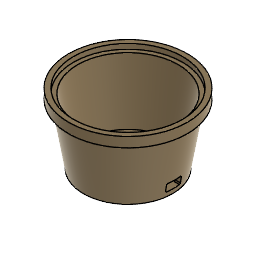
pot bottom v2 (Autodesk Fusion 360 design; units mm, degrees)
Autodesk Fusion 360 part; units mm, degrees
sketch "Sketch1" plane through (0, 0, 0) normal (0, 1, 0) x (1, 0, 0)
  line L0 (0, 0) -> (0, -70)
  line L1 (0, -70) -> (60, -70)
  line L2 (60, -70) -> (60, -60)
  line L3 (60, -60) -> (55, -60)
  line L4 (55, -60) -> (45, 0)
  line L5 (45, 0) -> (0, 0)
  dimension "d1" = 90
  dimension "d2" = 70
  dimension "d3" = 45
  dimension "d4" = 60
  dimension "d5" = 5
  dimension "d6" = 10
  constraint coincident L0.start L5.end
  constraint vertical L0
  constraint perpendicular L0 L1
  constraint perpendicular L1 L2
  constraint perpendicular L2 L3
  measures "d1" angle of L0 L5
  measures "d2" distance of L0.start L0.end
  measures "d3" distance of L0.start L4.end
  measures "d4" distance of L0.end L1.end
  measures "d5" distance of L2.end L3.end
  measures "d6" distance of L1.end L2.end
revolve "Revolve1" add sketch "Sketch1" angle 360 about axis through (0, 0, 0) along (0, 0, 1)
shell "Shell1" thickness 5 removed faces 1 at (28.282, -12.1475, 70)
sketch "Sketch2" plane through (0, 0, 0) normal (1, 0, 0) x (0, 1, 0)
  line L0 (-7.5, 13) -> (7.5, 13)
  line L1 (7.5, 13) -> (7.5, 5)
  line L2 (7.5, 5) -> (-7.5, 5)
  line L3 (-7.5, 5) -> (-7.5, 13)
  dimension "d9" = 5
  dimension "d10" = 15
  dimension "d11" = 8
  dimension "d12" = 7.5
  constraint horizontal L0
  constraint vertical L1
  constraint horizontal L2
  constraint vertical L3
  measures "d9" distance of origin L2
  measures "d10" distance of L0.start L0.end
  measures "d11" distance of L0.end L1.end
  measures "d12" distance of origin L1
extrude "Extrude1" cut sketch "Sketch2" along normal through all
fillet "Fillet1" radius 1 4 edges at (42.642, 7.5, 5) (43.9954, 7.5, 13) (42.642, -7.5, 5) (43.9954, -7.5, 13)
